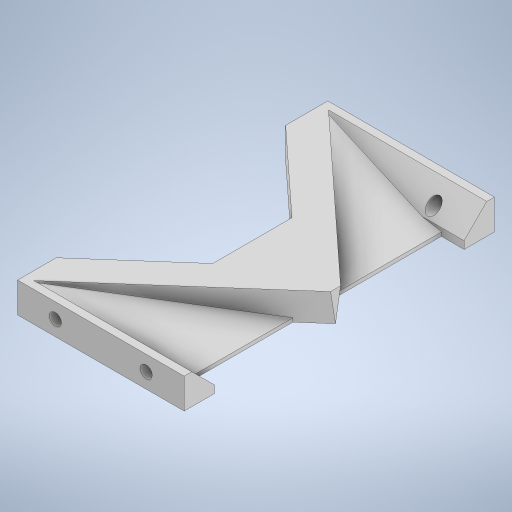
# Autodesk Inventor part: chest_cover
Saved by Autodesk Inventor 2024.1 (Build 281209000, 209)
## iProperties
Created: 2024-03-02
Part Number: chest_cover
Material: 一般
Document SubType Name: Modeling
Designer: hibik
Density: 1 g/cm^3
Appearance: 既定
Author: hibik
Autodesk Inventor part; units mm, degrees
ref_plane "YZ Plane" through (0, 0, 0) normal (1, 0, 0) x (0, 1, 0)
ref_plane "XZ Plane" through (0, 0, 0) normal (0, 1, 0) x (-1, 0, 0)
sketch "スケッチ1" plane through (0, 0, 0) normal (0, 1, 0) x (-1, 0, 0)
  line L0 (22, 0) -> (0, 0)
  line L1 (0, 0) -> (0, -41)
  line L2 (0, -41) -> (22, -41)
  line L3 (22, -41) -> (22, 0)
  dimension "d0" = 41
  dimension "d1" = 22
  constraints: 8 end point, 2 parallel, 1 coincident, 1 horizontal, 1 perpendicular
  measures "d0" distance of L2.end L0.start
  measures "d1" distance of L0.start L0.end
extrude "押し出し1" add sketch "スケッチ1" along normal blind 4
sketch "スケッチ2" plane through (0, 0, 0) normal (1, 0, 0) x (0, 0, -1)
  line L0 (0, 0) -> (41, 0) projected
  line L1 (41, 0) -> (41, 4) projected
  line L2 (0, 4) -> (41, 4) projected
  line L3 (0, 0) -> (0, 4) projected
  point P0 (20, 0)
  constraints: 1 point on line
ref_plane "作業平面1" through (-22, 4, 0) normal (0.1788854, 0.9838699, 0) x (0.7333333, -0.1333333, -0.6666667)
sketch "スケッチ3" plane through (-22, 4, 0) normal (0.1788854, 0.9838699, 0) x (0.7333333, -0.1333333, -0.6666667)
  line L0 (27.3333, 30.5596) -> (0, 0) projected
  line L1 (16.6667, -14.9071) -> (44, 15.6525) projected
  line L2 (16.6667, -14.9071) -> (44, 15.6525) projected
  line L3 (0, 0) -> (30, 0)
  line L4 (27.3333, 30.5596) -> (30, 0)
  line L5 (-20, -21.3606) -> (60, -21.3606)
  line L6 (60, -21.3606) -> (60, 40)
  line L7 (60, 40) -> (-20, 40)
  line L8 (-20, 40) -> (-20, -21.3606)
  line L9 (16.6667, -14.9071) -> (19.3333, -11.9257)
  line L10 (19.3333, -11.9257) -> (2.6667, 2.9814)
  line L11 (2.6667, 2.9814) -> (0, 0)
  line L12 (0, 0) -> (16.6667, -14.9071)
  line L13 (44, 15.6525) -> (41.3333, 12.6711)
  line L14 (41.3333, 12.6711) -> (24.6667, 27.5782)
  line L15 (24.6667, 27.5782) -> (27.3333, 30.5596)
  line L16 (27.3333, 30.5596) -> (44, 15.6525)
  point P0 (41.3333, 12.6711)
  point P1 (27.8413, 24.7387)
  point P2 (6, 0)
  dimension "d10" = 4
  dimension "d11" = 4
  constraints: 28 end point, 6 parallel, 4 point on line, 3 perpendicular, 2 horizontal
  measures "d10" distance between parallel lines of L12 L10
  measures "d11" distance between parallel lines of L16 L14
extrude "押し出し2" cut sketch "スケッチ3" along normal through all contours L14 L1 L4 | L1 L10 L3 | L8 L7 L6 L5
sketch "スケッチ4" plane through (0, 4, 0) normal (0, 1, 0) x (1, 0, 0)
  line L0 (0, 20.672) -> (-17.671, 37) projected
  line L1 (-22, 41) -> (-22, 0) projected
  line L2 (-17.4545, 4) -> (0, 19.36) projected
  line L3 (0, 19.36) -> (0, 20.672) projected
  line L4 (-22, 5.0983) -> (-11, 14.7783)
  line L5 (-11, 14.7783) -> (-11, 25.2537)
  line L6 (-11, 25.2537) -> (-22, 35.4177)
  line L7 (-22, 0) -> (0, 19.36) projected
  line L8 (0, 20.672) -> (-22, 41) projected
  line L9 (0, 4) -> (-17.4545, 4) projected
  line L10 (-17.671, 37) -> (0, 37) projected
  line L11 (0, 37) -> (0, 41) projected
  line L12 (0, 41) -> (-22, 41) projected
  line L13 (-22, 0) -> (0, 0) projected
  line L14 (0, 0) -> (0, 4) projected
  point P0 (-11, 20.016)
  point P1 (0, 20.016)
  dimension "d6" = 11
  dimension "d7" = 3.8274
  constraints: 6 end point, 2 midpoint, 2 parallel, 2 point on line, 1 horizontal alignment, 1 vertical
  measures "d6" distance between parallel lines of L3 L5
  measures "d7" distance between parallel lines of L2 L4
extrude "押し出し3" cut sketch "スケッチ4" against normal through all contours L6 L5 L4 L1
chamfer "面取り1" distance 3 angle 45 2 edges at (-8.7273, 4, -4) (-8.8355, 4, -37)
chamfer "面取り2" distance 3 angle 45 1 edges at (0, 0, -12)
chamfer "面取り3" distance 3 angle 45 1 edges at (0, 0, -28.5)
sketch "スケッチ5" plane through (0, 0, -41) normal (0, 0, -1) x (-1, 0, 0)
  circle A0 centre (5, 2) radius 0.8
  circle A1 centre (17, 2) radius 0.8
  line L0 (0, 0) -> (0, 4) projected
  line L1 (22, 0) -> (22, 4) projected
  point P0 (0, 2)
  dimension "d21" = 1.6
  dimension "d22" = 1.6
  dimension "d23" = 5
  dimension "d24" = 5
  constraints: 2 centre point, 2 horizontal alignment, 1 midpoint
  measures "d21" diameter of A0
  measures "d22" diameter of A1
  measures "d23" distance from line of L0 A0.centre
  measures "d24" distance from line of L1 A1.centre
extrude "押し出し4" cut sketch "スケッチ5" against normal up to surface surface through (-5.5, 2.5, -38.5) normal (0, 0.7071068, 0.7071068)
sketch "スケッチ7" plane through (-22, 0, 0) normal (0, 0, 1) x (1, 0, 0)
  circle A0 centre (17, 2) radius 0.8 projected
  circle A1 centre (5, 2) radius 0.8 projected
  point P0 (22, 0)
extrude "押し出し5" cut sketch "スケッチ7" against normal up to surface surface through (-14.3, 2.5, -2.5) normal (0, 0.7071068, -0.7071068)
equation "\"d11\" = d10"
equation "\"d24\" = d23"
